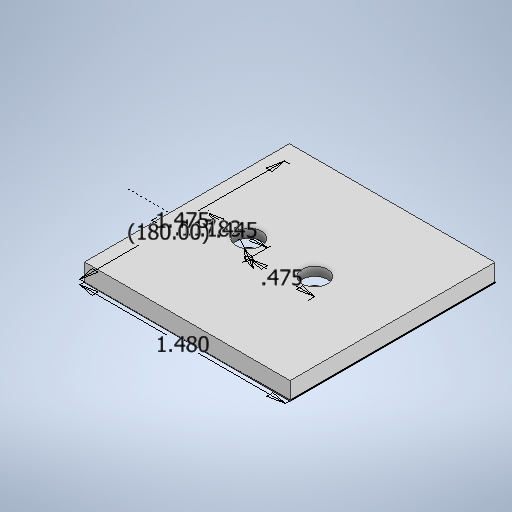
# Autodesk Inventor part: gps sensor holder
Saved by Autodesk Inventor 2025.1 (Build 291241020, 241B)
## iProperties
Created: 2025-01-09
Part Number: gps sensor holder
Material: Generic
Document SubType Name: Modeling
Designer: AtuStem
Density: 1 g/cm^3
Appearance: Default
Author: AtuStem
Autodesk Inventor part; units mm, degrees
ref_plane "YZ Plane" through (0, 0, 0) normal (1, 0, 0) x (0, 1, 0)
ref_plane "XZ Plane" through (0, 0, 0) normal (0, 1, 0) x (-1, 0, 0)
ref_plane "XY Plane" through (0, 0, 0) normal (0, 0, 1) x (1, 0, 0)
sketch "Sketch1" plane through (0, 0, 0) normal (0, 1, 0) x (-1, 0, 0)
  line L0 (0, 0) -> (37.592, 0)
  line L1 (37.592, 0) -> (37.592, 37.465)
  line L2 (37.592, 37.465) -> (0, 37.465)
  line L3 (0, 37.465) -> (0, 0)
  line L4 (37.592, 18.7325) -> (26.289, 18.7325)
  line L5 (37.592, 18.7325) -> (48.895, 18.7325) construction
  circle A0 centre (26.289, 18.7325) radius 2.3241
  circle A1 centre (14.224, 18.7325) radius 2.3241
  line L6 (34.6202, 34.4932) -> (34.6202, 2.9718)
  line L7 (34.6202, 2.9718) -> (2.9718, 2.9718)
  line L8 (2.9718, 2.9718) -> (2.9718, 34.4932)
  line L9 (2.9718, 34.4932) -> (34.6202, 34.4932)
  dimension "d0" = 37.592
  dimension "d1" = 37.465
  dimension "d2" = 11.303
  dimension "d3" = 180
  dimension "d4" = 4.6482
  dimension "d7" = 12.065
  dimension "d14" = 2.9718
  constraints: 20 end point, 4 horizontal, 4 parallel, 2 centre point, 2 perpendicular, 1 coincident, 1 collinear, 1 midpoint, 5 other
  measures "d0" distance of L2.end L1.end
  measures "d1" distance of L1.end L0.end
  measures "d2" distance of L4.start L4.end
  measures "d3" angle of L4 L5
  measures "d4" diameter of A0
  measures "d7" distance of A0.centre A1.centre
  measures "d14" distance between parallel lines of L1 L6
extrude "Extrusion1" add sketch "Sketch1" along normal blind 3.175 contours L6 L7 L8 L9 | L3 L2 L1 L0
extrude "Extrusion2" cut sketch "Sketch1" along normal blind 1.5875 contours L6 L7 L8 L9
body "Solid1"
